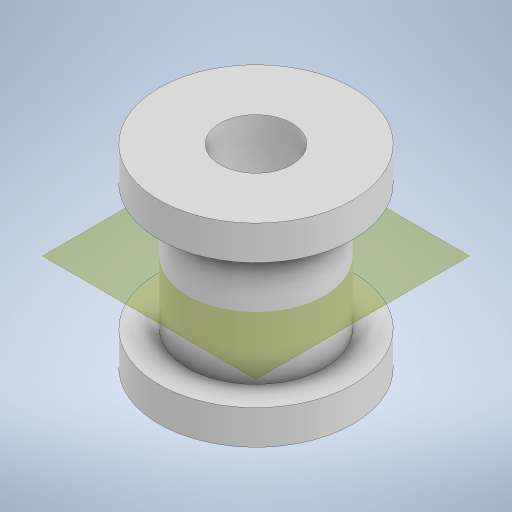
# Autodesk Inventor part: Belt tensor2
Saved by Autodesk Inventor 2023 (Build 270158000, 158)
## iProperties
Created: 2020-10-03
Part Number: Belt tensor2
Material: Generic
Document SubType Name: Modeling
Designer: ferrerx
Density: 1 g/cm^3
Appearance: Default
Author: ferrerx
Autodesk Inventor part; units mm, degrees
ref_plane "YZ Plane" through (0, 0, 0) normal (1, 0, 0) x (0, 1, 0)
ref_plane "XZ Plane" through (0, 0, 0) normal (0, 1, 0) x (-1, 0, 0)
ref_plane "XY Plane" through (0, 0, 0) normal (0, 0, 1) x (1, 0, 0)
sketch "Sketch1" plane through (0, 0, 0) normal (0, 1, 0) x (-1, 0, 0)
  circle A0 centre (0, 0) radius 3.15
  circle A1 centre (0, 0) radius 6
  dimension "d0" = 6.3
  dimension "d2" = 12
  constraints: 2 centre point, 2 coincident
  measures "d0" diameter of A0
  measures "d2" diameter of A1
extrude "Extrusion1" add sketch "Sketch1" along normal blind 14
sketch "Sketch2" plane through (0, 14, 0) normal (0, 1, 0) x (1, 0, 0)
  circle A0 centre (0, 0) radius 2.6288
  circle A1 centre (0, 0) radius 3.15 projected
  circle A2 centre (0, 0) radius 8.5
  dimension "d5" = 17
  constraints: 2 centre point, 2 coincident
  measures "d5" diameter of A2
extrude "Extrusion2" add sketch "Sketch2" against normal blind 3 contours A2
ref_plane "Work Plane1" through (0, 5.5, 0) normal (0, -1, 0) x (1, 0, 0)
mirror "Mirror1" about plane through (0, 5.5, 0) normal (0, -1, 0) of "Extrusion2"
ref_plane "Work Plane2" through (0, 5.5, 0) normal (0, -1, 0) x (1, 0, 0)
body "Solid1"
